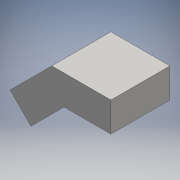
# Autodesk Inventor part: Orthogonal Bracket
Saved by Autodesk Inventor 2016 (Build 200138000, 138)
## iProperties
Created: 2015-12-30
Part Number: Orthogonal Bracket
Material: Generic
Document SubType Name: Modeling
Designer: jonathan
Density: 1 g/cm^3
Appearance: Default
Author: jonathan
Autodesk Inventor part; units mm, degrees
ref_plane "YZ Plane" through (0, 0, 0) normal (1, 0, 0) x (0, 1, 0)
ref_plane "XZ Plane" through (0, 0, 0) normal (0, 1, 0) x (-1, 0, 0)
ref_plane "XY Plane" through (0, 0, 0) normal (0, 0, 1) x (1, 0, 0)
sketch "Sketch1" plane through (0, 0, 0) normal (0, 1, 0) x (-1, 0, 0)
  line L0 (0, 0) -> (0, -10)
  line L1 (0, -10) -> (15.8579, -10)
  line L2 (15.8579, -10) -> (27.0711, -21.2132)
  line L3 (27.0711, -21.2132) -> (34.1421, -14.1421)
  line L4 (34.1421, -14.1421) -> (20, 0)
  line L5 (20, 0) -> (0, 0)
  line L6 (20, 0) -> (15.8579, -10)
  line L7 (15.8579, -10) -> (13.3455, -10)
  dimension "d0" = 20
  dimension "d6" = 10
  dimension "d10" = 45
  constraints: 16 end point, 2 equal length, 2 parallel, 2 perpendicular, 1 point on line, 1 vertical
  measures "d0" distance of L4.end L0.start
  measures "d6" distance of L0.start L0.end
  measures "d10" angle of L5 L3
extrude "Extrusion1" add sketch "Sketch1" along normal blind 20
body "Solid1"
